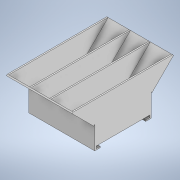
# Autodesk Inventor part: BeadCompartments_2
Saved by Autodesk Inventor 2020 (Build 240168000, 168)
## iProperties
Created: 2021-12-09
Part Number: BeadCompartments_2
Material: Generic
Document SubType Name: Modeling
Designer: danie
Density: 1 g/cm^3
Appearance: Default
Author: danie
Autodesk Inventor part; units mm, degrees
ref_plane "YZ Plane" through (0, 0, 0) normal (1, 0, 0) x (0, 1, 0)
ref_plane "XZ Plane" through (0, 0, 0) normal (0, 1, 0) x (-1, 0, 0)
ref_plane "XY Plane" through (0, 0, 0) normal (0, 0, 1) x (1, 0, 0)
sketch "Sketch1" plane through (0, 0, 0) normal (0, 1, 0) x (-1, 0, 0)
  line L0 (0, 0) -> (-152.4, 0)
  line L1 (-152.4, 0) -> (-152.4, -127)
  line L2 (-152.4, -127) -> (0, -127)
  line L3 (0, -127) -> (0, 0)
  line L4 (0, 0) -> (-152.4, 0)
  line L5 (-152.4, 0) -> (-152.4, 3.175)
  line L6 (-152.4, 3.175) -> (0, 3.175)
  line L7 (0, 3.175) -> (0, 0)
  line L8 (0, -127) -> (-152.4, -127)
  line L9 (-152.4, -127) -> (-152.4, -130.175)
  line L10 (-152.4, -130.175) -> (0, -130.175)
  line L11 (0, -130.175) -> (0, -127)
  dimension "d0" = 152.4
  dimension "d1" = 127
  dimension "d2" = 152.4
  dimension "d3" = 3.175
  dimension "d4" = 152.4
  dimension "d5" = 3.175
  constraints: 24 end point, 6 parallel, 3 horizontal, 3 perpendicular
  measures "d0" distance of L2.end L1.end
  measures "d1" distance of L1.end L0.end
  measures "d2" distance of L5.end L6.end
  measures "d3" distance of L4.end L5.end
  measures "d4" distance of L10.end L9.end
  measures "d5" distance of L9.end L8.end
extrude "Extrusion1" add sketch "Sketch1" along normal blind 50.8 contours L0 L5 L6 L7 | L11 L10 L9 L2
sketch "Sketch2" plane through (0, 50.8, 0) normal (0, 1, 0) x (1, 0, 0)
  line L0 (0, -3.175) -> (152.4, -3.175) projected
  line L1 (0, -3.175) -> (-3.175, -3.175)
  line L2 (-3.175, -3.175) -> (-3.175, 130.175)
  line L3 (-3.175, 130.175) -> (0, 130.175)
  line L4 (0, 130.175) -> (0, -3.175)
  point P0 (0, 0)
  dimension "d8" = 3.175
  dimension "d9" = 133.35
  constraints: 8 end point, 2 parallel, 1 horizontal, 1 perpendicular
  measures "d8" distance of L2.end L3.end
  measures "d9" distance of L1.end L2.end
extrude "Extrusion2" add sketch "Sketch2" against normal blind 45.72
sketch "Sketch3" plane through (0, 0, 3.175) normal (0, 0, 1) x (1, 0, 0)
  line L0 (-3.175, 5.08) -> (0, 5.08) projected
  line L1 (-3.175, 5.08) -> (0, 5.08)
  line L2 (0, 5.08) -> (0, 0)
  line L3 (0, 0) -> (-3.175, 0)
  line L4 (-3.175, 0) -> (-3.175, 5.08)
  constraints: 8 end point, 2 parallel, 1 horizontal, 1 perpendicular
extrude "Extrusion3" add sketch "Sketch3" against normal blind 3.175
sketch "Sketch4" plane through (152.4, 0, -130.175) normal (0, 0, -1) x (-1, 0, 0)
  line L0 (152.4, 0) -> (155.575, 0)
  line L1 (155.575, 0) -> (155.575, 5.08)
  line L2 (155.575, 5.08) -> (152.4, 5.08)
  line L3 (152.4, 5.08) -> (152.4, 0)
  constraints: 8 end point, 2 parallel, 1 horizontal, 1 perpendicular
extrude "Extrusion4" add sketch "Sketch4" against normal blind 3.175
sketch "Sketch5" plane through (0, 50.8, 0) normal (0, 1, 0) x (1, 0, 0)
  line L0 (152.4, -3.175) -> (152.4, 0) projected
  line L1 (0, 127) -> (152.4, 127) projected
  line L2 (152.4, 0) -> (149.225, 0)
  line L3 (149.225, 0) -> (149.225, 127)
  line L4 (149.225, 127) -> (152.4, 127)
  line L5 (152.4, 127) -> (152.4, 0)
  point P0 (0, 0)
  dimension "d16" = 3.175
  constraints: 8 end point, 2 parallel, 1 horizontal, 1 perpendicular, 1 point on line
  measures "d16" distance of L3.end L4.end
extrude "Extrusion5" add sketch "Sketch5" against normal blind 45.72
sketch "Sketch7" plane through (0, 0, 0) normal (0, -1, 0) x (1, 0, 0)
  line L0 (-3.175, 3.175) -> (-3.175, 0) projected
  line L1 (152.4, -127) -> (152.4, 0) projected
  line L2 (-3.175, 3.175) -> (152.4, 3.175)
  line L3 (152.4, 3.175) -> (152.4, -9.525)
  line L4 (152.4, -9.525) -> (-3.175, -9.525)
  line L5 (-3.175, -9.525) -> (-3.175, 3.175)
  line L6 (-3.175, -130.175) -> (-3.175, 3.175) projected
  line L7 (-3.175, -130.175) -> (152.4, -130.175)
  line L8 (152.4, -130.175) -> (152.4, -117.475)
  line L9 (152.4, -117.475) -> (-3.175, -117.475)
  line L10 (-3.175, -117.475) -> (-3.175, -130.175)
  point P0 (0, 0)
  point P1 (-3.175, -117.475)
  dimension "d19" = 12.7
  dimension "d20" = 155.575
  dimension "d21" = 12.7
  constraints: 16 end point, 4 parallel, 2 horizontal, 2 perpendicular, 1 point on line
  measures "d19" distance of L2.end L3.end
  measures "d20" distance of L9.end L8.end
  measures "d21" distance of L8.end L7.end
extrude "Extrusion6" add sketch "Sketch7" along normal blind 3.175 contours L2 L3 L1 L4 L5 L0 | L9 L1 L8 L7 L6
sketch "Sketch8" plane through (0, 50.8, 0) normal (0, 1, 0) x (1, 0, 0)
  line L0 (0, 0) -> (49.53, 0) construction
  line L1 (49.53, 0) -> (49.53, 127) construction
  line L2 (49.53, 127) -> (0, 127) construction
  line L3 (0, 127) -> (0, 0) construction
  line L4 (149.225, 0) -> (152.4, 0) construction
  line L5 (149.225, 0) -> (99.695, 0) construction
  line L6 (99.695, 0) -> (99.695, 127) construction
  line L7 (99.695, 127) -> (149.225, 127) construction
  line L8 (149.225, 127) -> (149.225, 0) construction
  line L9 (99.695, 0) -> (96.52, 0)
  line L10 (96.52, 0) -> (96.52, 127)
  line L11 (96.52, 127) -> (99.695, 127)
  line L12 (99.695, 127) -> (99.695, 0)
  line L13 (49.53, 0) -> (52.705, 0)
  line L14 (52.705, 0) -> (52.705, 127)
  line L15 (52.705, 127) -> (49.53, 127)
  line L16 (49.53, 127) -> (49.53, 0)
  dimension "d24" = 49.53
  dimension "d25" = 127
  dimension "d26" = 49.53
  dimension "d27" = 127
  dimension "d28" = 3.175
  dimension "d29" = 127
  dimension "d30" = 3.175
  dimension "d31" = 127
  constraints: 32 end point, 8 parallel, 4 horizontal, 4 perpendicular
  measures "d24" distance of L2.end L1.end
  measures "d25" distance of L1.end L0.end
  measures "d26" distance of L6.end L7.end
  measures "d27" distance of L5.end L6.end
  measures "d28" distance of L10.end L11.end
  measures "d29" distance of L9.end L10.end
  measures "d30" distance of L15.end L14.end
  measures "d31" distance of L14.end L13.end
extrude "Extrusion7" add sketch "Sketch8" against normal blind 45.72
sketch "Sketch9" plane through (152.4, 50.8, 3.175) normal (1, 0, 0) x (0, 0, -1)
  line L0 (0, 0) -> (133.35, 0)
  line L1 (133.35, 0) -> (133.35, 50.8)
  line L2 (133.35, 50.8) -> (0, 50.8)
  line L3 (0, 50.8) -> (0, 0)
  line L4 (133.35, 50.8) -> (184.15, 50.8)
  line L5 (184.15, 50.8) -> (133.35, 0)
  line L6 (0, 50.8) -> (-50.8, 50.8)
  line L7 (0, 50.8) -> (50.8, 50.8) construction
  line L8 (-50.8, 50.8) -> (0, 0)
  point P0 (3.175, -50.8)
  dimension "d34" = 133.35
  dimension "d35" = 50.8
  dimension "d36" = 50.8
  dimension "d37" = 50.8
  dimension "d38" = 180
  constraints: 18 end point, 3 equal length, 3 horizontal, 1 collinear, 1 perpendicular
  measures "d34" distance of L2.end L1.end
  measures "d35" distance of L1.end L0.end
  measures "d36" distance of L1.end L4.end
  measures "d37" distance of L2.end L6.end
  measures "d38" angle of L6 L7
extrude "Extrusion8" add sketch "Sketch9" against normal blind 3.175
sketch "Sketch10" plane through (-3.175, 50.8, -130.175) normal (-1, 0, 0) x (0, 0, 1)
  line L0 (3.175, 0) -> (0, 0) projected
  line L1 (0, 0) -> (133.35, 0)
  line L2 (133.35, 0) -> (133.35, 50.8)
  line L3 (133.35, 50.8) -> (0, 50.8)
  line L4 (0, 50.8) -> (0, 0)
  line L5 (-50.8, 50.8) -> (184.15, 50.8) projected
  line L6 (0, 50.8) -> (-50.8, 50.8)
  line L7 (-50.8, 50.8) -> (0, 0)
  line L8 (133.35, 50.8) -> (184.15, 50.8)
  line L9 (133.35, 0) -> (184.15, 50.8)
  point P0 (130.175, -50.8)
  dimension "d41" = 133.35
  dimension "d42" = 50.8
  constraints: 16 end point, 2 parallel, 1 horizontal, 1 perpendicular
  measures "d41" distance of L3.end L2.end
  measures "d42" distance of L2.end L1.end
extrude "Extrusion9" add sketch "Sketch10" against normal blind 3.175
sketch "Sketch11" plane through (-3.175, 50.8, 3.175) normal (0, -0.7071, 0.7071) x (1, 0, 0)
  line L0 (0, 71.842) -> (0, -94.2927) projected
  line L1 (155.575, 0) -> (155.575, -38.1661) projected
  line L2 (0, 71.842) -> (155.575, 71.842)
  line L3 (155.575, 71.842) -> (155.575, 0)
  line L4 (155.575, 0) -> (0, 0)
  line L5 (0, 0) -> (0, 71.842)
  point P0 (3.175, -38.1661)
  point P1 (0, 0)
  constraints: 8 end point, 2 parallel, 1 horizontal, 1 perpendicular
extrude "Extrusion10" add sketch "Sketch11" along normal blind 3.175
sketch "Sketch12" plane through (152.4, 50.8, -130.175) normal (0, -0.7071, -0.7071) x (-1, 0, 0)
  line L0 (0, 0) -> (0, 71.842) projected
  line L1 (152.4, 0) -> (155.575, 0) projected
  line L2 (0, 71.842) -> (155.575, 71.842)
  line L3 (155.575, 71.842) -> (155.575, 0)
  line L4 (155.575, 0) -> (0, 0)
  line L5 (0, 0) -> (0, 71.842)
  point P0 (152.4, -127.9686)
  constraints: 8 end point, 2 parallel, 1 horizontal, 1 perpendicular
extrude "Extrusion11" add sketch "Sketch12" along normal blind 3.175
sketch "Sketch13" plane through (-3.175, 101.6, 53.975) normal (0, 1, 0) x (1, 0, 0)
  line L0 (52.705, 180.975) -> (52.705, 53.975) construction
  line L1 (52.705, 53.975) -> (52.705, 0) construction
  line L2 (152.4, 0) -> (3.175, 0) construction
  line L3 (55.88, 53.975) -> (55.88, 180.975) construction
  line L4 (55.88, 180.975) -> (55.88, 234.95) construction
  line L5 (3.175, 234.95) -> (152.4, 234.95) construction
  line L6 (52.705, 0) -> (55.88, 0)
  line L7 (55.88, 0) -> (55.88, 234.95)
  line L8 (55.88, 234.95) -> (52.705, 234.95)
  line L9 (52.705, 234.95) -> (52.705, 0)
  point P0 (3.175, 53.975)
  constraints: 12 end point, 3 parallel, 2 point on line, 1 horizontal, 1 perpendicular, 1 vertical
extrude "Extrusion12" add sketch "Sketch13" against normal blind 3.175
sketch "Sketch14" plane through (52.705, 101.6, 53.975) normal (1, 0, 0) x (0, 0, -1)
  line L0 (3.175, -3.175) -> (50.8, -50.8)
  line L1 (50.8, -50.8) -> (50.8, -3.175)
  line L2 (231.775, -3.175) -> (3.175, -3.175) projected
  point P0 (53.975, -101.6)
  constraints: 4 end point, 1 point on line
extrude "Extrusion13" add sketch "Sketch14" against normal blind 3.175
sketch "Sketch15" plane through (52.705, 101.6, 53.975) normal (1, 0, 0) x (0, 0, -1)
  line L0 (50.8, -50.8) -> (50.8, -3.175) projected
  line L1 (50.8, -3.175) -> (184.15, -3.175)
  line L2 (184.15, -3.175) -> (184.15, -50.8)
  line L3 (184.15, -50.8) -> (50.8, -50.8)
  line L4 (50.8, -50.8) -> (50.8, -3.175)
  line L5 (184.15, -50.8) -> (231.775, -3.175)
  line L6 (231.775, -3.175) -> (184.15, -3.175)
  line L7 (231.775, -3.175) -> (50.8, -3.175) projected
  point P0 (53.975, -101.6)
  constraints: 12 end point, 2 parallel, 1 collinear, 1 horizontal, 1 perpendicular
extrude "Extrusion14" add sketch "Sketch15" against normal blind 3.175
sketch "Sketch16" plane through (-3.175, 101.6, 53.975) normal (0, 1, 0) x (1, 0, 0)
  line L0 (152.4, 53.975) -> (102.87, 53.975) construction
  line L1 (102.87, 53.975) -> (102.87, 0) construction
  line L2 (152.4, 0) -> (55.88, 0) construction
  line L3 (55.88, 180.975) -> (99.695, 180.975) construction
  line L4 (99.695, 180.975) -> (99.695, 234.95) construction
  line L5 (55.88, 234.95) -> (152.4, 234.95) construction
  line L6 (102.87, 0) -> (99.695, 0)
  line L7 (99.695, 0) -> (99.695, 234.95)
  line L8 (99.695, 234.95) -> (102.87, 234.95)
  line L9 (102.87, 234.95) -> (102.87, 0)
  point P0 (3.175, 53.975)
  constraints: 12 end point, 3 parallel, 2 point on line, 1 horizontal, 1 perpendicular, 1 vertical
extrude "Extrusion15" add sketch "Sketch16" against normal blind 3.175
sketch "Sketch17" plane through (99.695, 101.6, 53.975) normal (1, 0, 0) x (0, 0, -1)
  line L0 (231.775, -3.175) -> (3.175, -3.175) projected
  line L1 (3.175, -3.175) -> (50.8, -50.8)
  line L2 (50.8, -50.8) -> (50.8, -3.175)
  line L3 (50.8, -3.175) -> (3.175, -3.175)
  line L4 (50.8, -3.175) -> (184.15, -3.175)
  line L5 (184.15, -3.175) -> (184.15, -50.8)
  line L6 (184.15, -50.8) -> (50.8, -50.8)
  line L7 (50.8, -50.8) -> (50.8, -3.175)
  line L8 (184.15, -3.175) -> (231.775, -3.175)
  line L9 (184.15, -50.8) -> (231.775, -3.175)
  point P0 (53.975, -101.6)
  constraints: 18 end point, 2 horizontal, 2 parallel, 2 perpendicular, 1 vertical
extrude "Extrusion16" add sketch "Sketch17" against normal blind 3.175
body "Solid1"
